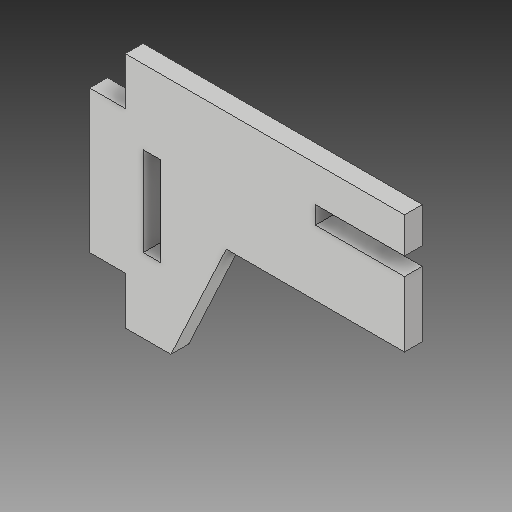
# Autodesk Inventor part: Camera bracket raiser
Saved by Autodesk Inventor 2018 (Build 220112000, 112)
## iProperties
Created: 2018-05-02
Part Number: Camera bracket raiser
Material: Generic
Document SubType Name: Modeling
Designer: Ajith Thomas
Density: 1 g/cm^3
Appearance: Default
Mass: 3.72222 g
Surface Area: 32.157 cm^2
Volume: 3.72222 cm^3
Author: Ajith Thomas
Autodesk Inventor part; units mm, degrees
ref_plane "YZ Plane" through (0, 0, 0) normal (1, 0, 0) x (0, 1, 0)
ref_plane "XZ Plane" through (0, 0, 0) normal (0, 1, 0) x (-1, 0, 0)
ref_plane "XY Plane" through (0, 0, 0) normal (0, 0, 1) x (1, 0, 0)
sketch "Sketch1" plane through (0, 0, 0) normal (0, 0, 1) x (1, 0, 0)
  line L0 (0, 0) -> (-15, 0) construction
  line L1 (0, 0) -> (0, 3) projected
  line L2 (-15, 3) -> (0, 3) construction
  line L3 (-15, 0) -> (-15, 3) construction
  line L4 (15, 0) -> (15, 3) projected
  line L5 (15, 9) -> (-15, 9)
  line L6 (-15, -11) -> (15, -11)
  line L7 (15, -11) -> (15, 9)
  line L8 (0, 3) -> (15, 3)
  line L9 (0, 0) -> (15, 0)
  line L10 (0, 3) -> (0, 0)
  line L11 (15, 3) -> (15, 0)
  line L12 (-15, 9) -> (-32, 9)
  line L13 (-32, 9) -> (-32, -31)
  line L14 (-15, -11) -> (-24.3262, -31)
  line L15 (-15, -11) -> (7.0676, -11) construction
  line L16 (-24.3262, -31) -> (-32, -31)
  line L17 (-32, 1) -> (-38, 1)
  line L18 (-38, 1) -> (-38, -23)
  line L19 (-38, -23) -> (-32, -23)
  line L20 (-32, -23) -> (-32, 1)
  dimension "d0" = 20
  dimension "d1" = 6
  dimension "d3" = 15
  dimension "d4" = 17
  dimension "d5" = 40
  dimension "d6" = 115
  dimension "d7" = 47
  dimension "d8" = 6
  dimension "d9" = 8
  dimension "d10" = 8
  constraints: 32 end point, 6 horizontal, 4 perpendicular, 3 parallel, 1 equal length, 1 point on line, 1 vertical
  measures "d0" distance of L6.start L5.end
  measures "d1" distance between parallel lines of L5 L2
  measures "d3" distance between parallel lines of L4 L1
  measures "d4" distance of L5.end L12.end
  measures "d5" distance of L12.end L13.end
  measures "d6" angle of L14 L15
  measures "d7" distance between parallel lines of L7 L20
  measures "d8" distance between parallel lines of L20 L18
  measures "d9" distance between parallel lines of L17 L12
  measures "d10" distance between parallel lines of L16 L19
extrude "Extrusion1" add sketch "Sketch1" along normal blind 3 contours L9 L7 L6 L14 L16 L13 L12 L5 L8 L1 | L13 L19 L18 L17
sketch "Sketch2" plane through (0, 0, 0) normal (0, 0, -1) x (-1, 0, 0)
  line L0 (26, -18.5) -> (29, -18.5)
  line L1 (29, -18.5) -> (29, -3.5)
  line L2 (29, -3.5) -> (26, -3.5)
  line L3 (26, -3.5) -> (26, -18.5)
  line L4 (-15, 9) -> (32, 9) projected
  line L5 (32, 9) -> (32, 1) projected
  point P0 (0, 0)
  dimension "d13" = 3
  dimension "d14" = 15
  dimension "d15" = 12.5
  dimension "d16" = 3
  constraints: 8 end point, 2 parallel, 1 horizontal, 1 perpendicular
  measures "d13" distance of L2.end L1.end
  measures "d14" distance of L1.end L0.end
  measures "d15" distance between parallel lines of L4 L2
  measures "d16" distance between parallel lines of L5 L1
extrude "Extrusion2" cut sketch "Sketch2" against normal blind 3
body "Solid1"
